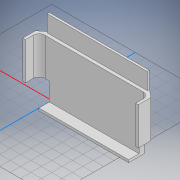
# Autodesk Inventor part: 000.001.009 - Накладка центральная
Saved by Autodesk Inventor 2022 (Build 260153000, 153)
## iProperties
Created: 2022-12-25
Part Number: 000.001.009 - Накладка центральная
Material: Типовые
Document SubType Name: Modeling
Designer: Ivan Petrov
Density: 1 g/cm^3
Appearance: По умолчанию
Author: Ivan Petrov
Autodesk Inventor part; units mm, degrees
ref_plane "YZ Plane" through (0, 0, 0) normal (1, 0, 0) x (0, 1, 0)
ref_plane "XZ Plane" through (0, 0, 0) normal (0, 1, 0) x (-1, 0, 0)
ref_plane "XY Plane" through (0, 0, 0) normal (0, 0, 1) x (1, 0, 0)
sketch "Эскиз1" plane through (0, 0, 0) normal (0, 0, 1) x (1, 0, 0)
  line L0 (5.3151, -72.5414) -> (177.8151, -72.5414) projected
  line L1 (177.8151, -152.5414) -> (177.8151, -32.5414) projected
  line L2 (5.3151, -152.5414) -> (5.3151, -32.5414) projected
  line L3 (5.3151, -32.5414) -> (-4.6849, -32.5414) projected
  line L4 (-49.9349, -32.5414) -> (-4.6849, -32.5414) projected
  line L5 (-19.4349, 12.1553) -> (-19.4349, 32.2619) projected
  line L6 (-19.4349, 12.1553) -> (-19.4349, 9.9586) projected
  line L7 (-19.4349, 37.5652) -> (-19.4349, 32.2619) projected
  line L8 (-19.4349, 37.5652) -> (-19.4349, 39.4586) projected
  line L9 (235.5651, 39.4586) -> (-52.4349, 39.4586) projected
  line L10 (177.8151, -32.5414) -> (187.8151, -32.5414) projected
  line L11 (233.0651, -32.5414) -> (187.8151, -32.5414) projected
  line L12 (202.5651, 9.9586) -> (202.5651, 12.1553) projected
  line L13 (202.5651, 12.1553) -> (202.5651, 32.2619) projected
  line L14 (202.5651, 32.2619) -> (202.5651, 37.5652) projected
  line L15 (202.5651, 37.5652) -> (202.5651, 39.4586) projected
  line L16 (202.5651, 12.1553) -> (202.5651, 32.2619) projected
  line L17 (202.5651, 12.1553) -> (202.5651, 32.2619) projected
  line L18 (-19.4349, 9.9586) -> (-19.4349, -32.5414)
  line L19 (202.5651, 9.9586) -> (202.5651, -32.5414)
  point P0 (0, 0)
  constraints: 4 end point, 2 vertical, 4 other
extrude "Выдавливание1" add sketch "Эскиз1" along normal blind 10
sketch "Эскиз7" plane through (0, 0, 10) normal (0, 0, 1) x (1, 0, 0)
  line L0 (-19.4349, 39.4586) -> (-19.4349, -32.5414) projected
  line L1 (-19.4349, -32.5414) -> (5.3151, -32.5414) projected
  line L2 (-19.4349, 39.4586) -> (-14.4349, 39.4586)
  line L3 (-14.4349, 39.4586) -> (-14.4349, -32.5414)
  line L4 (-14.4349, -32.5414) -> (-19.4349, -32.5414)
  line L5 (-19.4349, -32.5414) -> (-19.4349, 39.4586)
  line L6 (202.5651, -32.5414) -> (202.5651, 39.4586) projected
  line L7 (177.8151, -32.5414) -> (202.5651, -32.5414) projected
  line L8 (202.5651, 39.4586) -> (197.5651, 39.4586)
  line L9 (197.5651, 39.4586) -> (197.5651, -32.5414)
  line L10 (197.5651, -32.5414) -> (202.5651, -32.5414)
  line L11 (202.5651, -32.5414) -> (202.5651, 39.4586)
  point P0 (0, 0)
  point P1 (-19.4349, 9.9586)
  point P2 (5.3151, -32.5414)
  point P3 (202.5651, 9.9586)
  dimension "d13" = 5
  dimension "d14" = 5
  constraints: 16 end point, 4 parallel, 2 horizontal, 2 perpendicular, 4 other
  measures "d13" distance of L3.end L0.end
  measures "d14" distance of L6.start L9.end
extrude "Выдавливание6" add sketch "Эскиз7" along normal blind 26
sketch "Эскиз8" plane through (-19.4349, -32.5414, 0) normal (0, -1, 0) x (1, 0, 0)
  line L0 (-30.5, 36) -> (14.75, 0) projected
  line L1 (0, 0) -> (0, 36) projected
  line L2 (0, 0) -> (24.75, 0) projected
  line L3 (197.25, 0) -> (222, 0) projected
  line L4 (252.5, 36) -> (207.25, 0) projected
  line L5 (222, 0) -> (222, 36) projected
  point P0 (19.4349, 0)
  point P1 (0, 11.7348)
  point P2 (222, 11.7348)
extrude "Выдавливание7" cut sketch "Эскиз8" against normal through all
fillet "Сопряжение1" radius 11.5 2 edges at (-14.4349, 3.4586, 10) (197.5651, 3.4586, 10)
sketch "Эскиз9" plane through (-4.6849, 39.4586, 0) normal (0, 1, 0) x (1, 0, 0)
  line L0 (192.5, 0) -> (0, 0) projected
  line L1 (0, 0) -> (192.5, 0)
  line L2 (192.5, 0) -> (192.5, -4)
  line L3 (192.5, -4) -> (0, -4)
  line L4 (0, -4) -> (0, 0)
  point P0 (4.6849, 0)
  dimension "d20" = 4
  constraints: 8 end point, 2 parallel, 1 horizontal, 1 perpendicular
  measures "d20" distance between parallel lines of L0 L3
extrude "Выдавливание8" add sketch "Эскиз9" along normal blind 32
sketch "Эскиз10" plane through (0, 0, 10) normal (0, 0, 1) x (1, 0, 0)
  line L0 (5.3151, -72.5414) -> (177.8151, -72.5414) projected
  line L1 (177.8151, -72.5414) -> (177.8151, -32.5414) projected
  line L2 (5.3151, -72.5414) -> (177.8151, -72.5414)
  line L3 (177.8151, -72.5414) -> (177.8151, -67.5414)
  line L4 (177.8151, -67.5414) -> (5.3151, -67.5414)
  line L5 (5.3151, -67.5414) -> (5.3151, -72.5414)
  point P0 (0, 0)
  dimension "d23" = 5
  constraints: 8 end point, 2 parallel, 1 horizontal, 1 perpendicular, 1 point on line
  measures "d23" distance of L3.end L2.end
extrude "Выдавливание9" add sketch "Эскиз10" along normal blind 20
